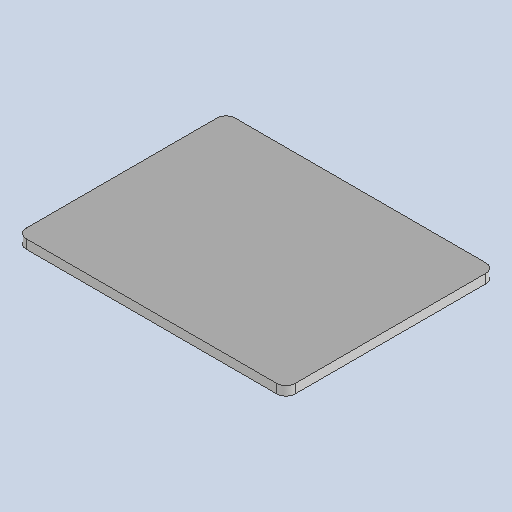
# Autodesk Inventor part: KND-1666 FDS 1000 CUP 1 01
Saved by Autodesk Inventor 2026.2 (Build 302298000, 298)
## iProperties
Created: 2025-06-24
Part Number: KND-1666 FDS 1000 CUP 1 01
Material: Stainless Steel
Document SubType Name: Sheet Metal
Designer: admin
Mass: 23.076 g
Surface Area: 31.7918 cm^2
Volume: 2.88451 cm^3
Density: 8 g/cm^3
Flat Pattern Width: 5.92 cm
Flat Pattern Length: 4.6 cm
Flat Pattern Area: 27.232 cm^2
Sheet Metal Rule: AISI304 2mm Die16
Sheet Metal Width: 59,200 mm
Sheet Metal Length: 46,000 mm
Sheet Metal Area: 2723,200 mm^2
Appearance: Default
Stock Number: Заглушка луча
Author: user
Autodesk Inventor part; units mm, degrees
ref_plane "YZ Plane" through (0, 0, 0) normal (1, 0, 0) x (0, 1, 0)
ref_plane "XZ Plane" through (0, 0, 0) normal (0, 1, 0) x (-1, 0, 0)
ref_plane "XY Plane" through (0, 0, 0) normal (0, 0, 1) x (1, 0, 0)
sketch "Sketch1" plane through (0, 0, 0) normal (0, 0, 1) x (1, 0, 0)
  line L0 (-29.6, -23) -> (29.6, -23)
  line L1 (29.6, -23) -> (29.6, 23)
  line L2 (29.6, 23) -> (-29.6, 23)
  line L3 (-29.6, 23) -> (-29.6, -23)
  line L4 (-29.6, -23) -> (29.6, 23) construction
  line L5 (29.6, -23) -> (-29.6, 23) construction
  point P0 (0, 0)
  point P1 (-29.6, 0)
  dimension "d154" = 59.2
  dimension "d155" = 46
  measures "d154" distance of L1.end L2.end
  measures "d155" distance of L0.end L1.end
extrude "Plate5" add sketch "Sketch1" along normal blind 2
fillet "Corner Round1" radius 2 4 edges at (29.6, 23, 1) (-29.6, 23, 1) (-29.6, -23, 1) (29.6, -23, 1)
derived "KND-1401 DrSysB DIMentions 01.ipt"
body "Solid3"
